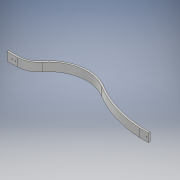
# Autodesk Inventor part: 8inch_Fin
Saved by Autodesk Inventor 2017 (Build 210142000, 142)
## iProperties
Created: 2016-05-03
Part Number: 8inch_Fin
Material: Generic
Document SubType Name: Modeling
Designer: Andres
Density: 1 g/cm^3
Appearance: Aluminum - Polished
Mass: 56.7968 g
Surface Area: 276.436 cm^2
Volume: 56.7968 cm^3
Author: Andres
Autodesk Inventor part; units mm, degrees
ref_plane "YZ Plane" through (0, 0, 0) normal (1, 0, 0) x (0, 1, 0)
ref_plane "XZ Plane" through (0, 0, 0) normal (0, 1, 0) x (-1, 0, 0)
ref_plane "XY Plane" through (0, 0, 0) normal (0, 0, 1) x (1, 0, 0)
sketch "Sketch1" plane through (0, 0, 0) normal (0, 0, 1) x (1, 0, 0)
  line L0 (0, 0) -> (150, 0)
  line L1 (150, 0) -> (150, 68)
  line L2 (150, 68) -> (0, 68)
  line L3 (0, 68) -> (0, 0)
  arc A0 (150, 51.1345) -> (0, 24.6854) centre (90, -47.1593) ccw
  line L4 (0, 24.6854) -> (150, 51.1345) construction
  line L5 (0, 24.6854) -> (152.314, 24.6854) construction
  arc A1 (-49, -0.0229) -> (0, 24.6854) centre (-51.433, 65.743) ccw
  arc A2 (150, 51.1345) -> (316.5, -0.0007) centre (333.3524, 351.5077) ccw
  line L6 (-49, -0.0229) -> (-80, -0.0229)
  line L7 (316.5, -0.0007) -> (341.5, -0.0007)
  line L8 (341.5, 4.9993) -> (316.6202, 4.9993)
  arc A3 (152.6051, 55.4022) -> (316.6202, 4.9993) centre (333.3524, 351.5077) ccw
  arc A4 (152.6051, 55.4022) -> (-3.9076, 27.8048) centre (90, -47.1593) ccw
  arc A5 (-49.0943, 4.9771) -> (-3.9076, 27.8048) centre (-51.433, 65.743) ccw
  line L9 (-49.0943, 4.9771) -> (-80, 4.9771)
  line L10 (-80, -0.0229) -> (-80, 4.9771)
  line L11 (341.5, -0.0007) -> (341.5, 4.9993)
  dimension "d0" = 150
  dimension "d1" = 68
  dimension "d2" = 10
  dimension "d3" = 90
  dimension "d4" = 65.8109
  dimension "d5" = 49
  dimension "d6" = 351.9122
  dimension "d7" = 166.5
  dimension "d8" = 31
  dimension "d9" = 25
  dimension "d10" = 5
  dimension "d11" = 5
  dimension "d12" = 5
  dimension "d31" = 30.9057
  constraints: 24 end point, 12 point on circle, 6 centre point, 4 horizontal, 3 tangent, 2 parallel, 2 point on line, 1 equal length, 1 perpendicular, 4 other
  measures "d0" distance of L1.end L2.end
  measures "d1" distance of L0.end L1.end
  measures "d2" angle of L5 L4
  measures "d3" horizontal distance of A0.centre L4.start
  measures "d4" radius of A1
  measures "d5" distance of L0.start L6.start
  measures "d6" radius of A2
  measures "d7" distance from line of L7.start L1
  measures "d8" distance of L6.start L6.end
  measures "d9" distance of L7.start L7.end
  measures "d10" radial gap between concentric circles of A1 A5
  measures "d11" distance of L9.end L6.end
  measures "d12" distance of L8.start L7.end
  measures "d31" distance of L9.start L9.end
extrude "Extrusion1" add sketch "Sketch1" along normal blind 25 contours A1 L6 L10 L9 A5 A4 L3 | L3 A4 L2 A0 | A0 L2 A4 L1 | L1 A4 A3 L8 L11 L7 A2 | L2 A4
sketch "Sketch7" plane through (-80, -0.0229, 0) normal (0, -1, 0) x (1, 0, 0)
  line L0 (31, 0) -> (31, 25) projected
  line L1 (421.5, 0) -> (421.5, 25) projected
  line L2 (0, 0) -> (0, 25) projected
  point P0 (80, 0)
  point P1 (25, 12.5)
  point P2 (15, 12.5)
  point P3 (31, 12.5)
  point P4 (31, 12.5)
  point P5 (416.5, 12.5)
  point P6 (421.5, 12.5)
  dimension "d44" = 5
  dimension "d52" = 25
  dimension "d53" = 15
  constraints: 3 horizontal alignment, 3 midpoint
  measures "d44" distance from line of L1 point (416.5, 12.5)
  measures "d52" distance from line of point (25, 12.5) L2
  measures "d53" distance from line of L2 point (15, 12.5)
hole "Hole2" at (-55, -0.0229, 12.5) at (-65, -0.0229, 12.5) at (336.5, -0.0229, 12.5) direction (0, 1, 0) diameter 2.642 end through all thread size "6-32 UNC" class "3B" standard "ANSI Unified Screw Threads"
body "Solid1"
